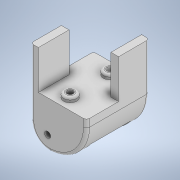
# Autodesk Inventor part: topMountThick
Saved by Autodesk Inventor 2020 (Build 240168000, 168)
## iProperties
Created: 2020-07-25
Part Number: topMountThick
Material: Generic
Document SubType Name: Modeling
Designer: PAB
Density: 1 g/cm^3
Appearance: Default
Author: PAB
Autodesk Inventor part; units mm, degrees
ref_plane "YZ Plane" through (0, 0, 0) normal (1, 0, 0) x (0, 1, 0)
ref_plane "XZ Plane" through (0, 0, 0) normal (0, 1, 0) x (-1, 0, 0)
ref_plane "XY Plane" through (0, 0, 0) normal (0, 0, 1) x (1, 0, 0)
sketch "Sketch1" plane through (0, 0, 0) normal (0, 1, 0) x (-1, 0, 0)
  line L0 (19.2, 20.5) -> (-17.2, 20.5)
  line L1 (-17.2, 20.5) -> (-17.2, -20.5)
  line L2 (-17.2, -20.5) -> (19.2, -20.5)
  line L3 (19.2, -20.5) -> (19.2, 20.5)
  point P0 (0, 0)
  dimension "d0" = 36.4
  dimension "d1" = 41
  constraints: 8 end point, 2 parallel, 1 horizontal, 1 perpendicular
  measures "d0" distance of L2.end L1.end
  measures "d1" distance of L1.end L0.end
extrude "Extrusion1" add sketch "Sketch1" along normal blind 5
sketch "Sketch2" plane through (0, 5, 0) normal (0, 1, 0) x (1, 0, 0)
  line L0 (-19.2, -20.5) -> (17.2, -20.5) projected
  line L1 (-19.2, -20.5) -> (-14.2, -20.5)
  line L2 (-14.2, -20.5) -> (-14.2, -0.5)
  line L3 (-14.2, -0.5) -> (-19.2, -0.5)
  line L4 (-19.2, -0.5) -> (-19.2, -20.5)
  line L5 (17.2, 20.5) -> (-19.2, 20.5) projected
  line L6 (17.2, 20.5) -> (12.2, 20.5)
  line L7 (12.2, 20.5) -> (12.2, 0.5)
  line L8 (12.2, 0.5) -> (17.2, 0.5)
  line L9 (17.2, 0.5) -> (17.2, 20.5)
  point P0 (0, 0)
  dimension "d4" = 5
  dimension "d5" = 20
  dimension "d6" = 5
  dimension "d7" = 20
  constraints: 16 end point, 4 parallel, 2 horizontal, 2 perpendicular
  measures "d4" distance of L3.end L2.end
  measures "d5" distance of L2.end L1.end
  measures "d6" distance of L8.end L7.end
  measures "d7" distance of L7.end L6.end
extrude "Extrusion2" add sketch "Sketch2" along normal blind 25.4
sketch "Sketch3" plane through (0, 5, 0) normal (0, 1, 0) x (1, 0, 0)
  circle A0 centre (-1, -13) radius 4.25
  circle A1 centre (-1, 13) radius 4.25
  line L0 (-14.2, -20.5) -> (-14.2, -0.5) projected
  line L1 (12.2, 20.5) -> (12.2, 0.5) projected
  point P0 (0, 0)
  dimension "d10" = 8.5
  dimension "d11" = 8.5
  dimension "d44" = 13.2
  dimension "d45" = 13.2
  constraints: 2 centre point
  measures "d10" diameter of A0
  measures "d11" diameter of A1
  measures "d44" distance from line of L0 A0.centre
  measures "d45" distance from line of L1 A1.centre
extrude "Extrusion3" add sketch "Sketch3" along normal blind 3
sketch "Sketch4" plane through (-1, 8, 13) normal (0, 1, 0) x (1, 0, 0)
  circle A0 centre (0, 0) radius 4.25 projected
  circle A1 centre (0, 0) radius 2
  circle A2 centre (0, 26) radius 4.25 projected
  circle A3 centre (0, 26) radius 2
  point P0 (1, 13)
  dimension "d14" = 4
  dimension "d15" = 4
  constraints: 2 centre point, 2 coincident
  measures "d14" diameter of A1
  measures "d15" diameter of A3
extrude "Extrusion4" cut sketch "Sketch4" against normal blind 10 contours A1 | A3
fillet "Fillet2" radius 1.5 2 edges at (-5.25, 8, -13) (-5.25, 8, 13)
sketch "Sketch5" plane through (0, 0, 0) normal (0, -1, 0) x (1, 0, 0)
  circle A0 centre (-1, 13) radius 2 projected
  circle A1 centre (-1, 13) radius 3
  circle A2 centre (-1, -13) radius 2 projected
  circle A3 centre (-1, -13) radius 3
  point P0 (0, 0)
  dimension "d20" = 6
  dimension "d21" = 6
  constraints: 2 centre point, 2 coincident
  measures "d20" diameter of A1
  measures "d21" diameter of A3
extrude "Extrusion5" cut sketch "Sketch5" against normal blind 3 contours A0 | A1 | A2 | A3
sketch "Sketch6" plane through (0, 0, 0) normal (0, -1, 0) x (1, 0, 0)
  line L0 (17.2, 20.5) -> (17.2, -20.5) projected
  line L1 (-19.2, -20.5) -> (-19.2, 20.5) projected
  line L2 (17.2, -20.5) -> (-19.2, -20.5)
  line L3 (-19.2, -20.5) -> (-19.2, 20.5)
  line L4 (-19.2, 20.5) -> (17.2, 20.5)
  line L5 (17.2, 20.5) -> (17.2, -20.5)
  point P0 (0, 0)
  constraints: 8 end point, 2 parallel, 1 horizontal, 1 perpendicular
extrude "Extrusion6" add sketch "Sketch6" along normal blind 25
sketch "Sketch7" plane through (0, -25, 0) normal (0, -1, 0) x (1, 0, 0)
  line L0 (-19.2, -13) -> (-4.2, -13)
  line L1 (-4.2, -13) -> (-4.2, -9.525)
  line L2 (-4.2, -9.525) -> (-19.2, -9.525)
  line L3 (-19.2, -9.525) -> (-19.2, -13)
  point P0 (0, 0)
  dimension "d26" = 15
  constraints: 8 end point, 2 parallel, 1 horizontal, 1 perpendicular
  measures "d26" distance of L2.end L1.end
extrude "Extrusion7" cut sketch "Sketch7" against normal blind 15
sketch "Sketch8" plane through (-19.2, -25, -13) normal (0, 0, 1) x (1, 0, 0)
  circle A0 centre (11, 9) radius 15.5
  point P0 (19.2, 25)
  dimension "d29" = 31
  constraints: 1 centre point
  measures "d29" diameter of A0
extrude "Extrusion8" cut sketch "Sketch8" along normal blind 26
sketch "Sketch9" plane through (-19.2, -25, -13) normal (0, 0, 1) x (1, 0, 0)
  arc A0 (23.6194, 0) -> (0, 19.9202) centre (11, 9) ccw projected
  circle A1 centre (11, 9) radius 2
  point P0 (19.2, 25)
  dimension "d32" = 4
  constraints: 1 centre point, 1 coincident
  measures "d32" diameter of A1
extrude "Extrusion9" cut sketch "Sketch9" against normal mid plane 100
fillet "Fillet3" radius 25 1 edges at (17.2, -25, 0)
fillet "Fillet4" radius 3 1 edges at (6.6653, -20.3901, 0)
fillet "Fillet5" radius 12 2 edges at (-19.2, -25, -16.75) (-19.2, -25, 16.75)
fillet "Fillet6" radius 2 1 edges at (-19.2, -5.0798, 0)
fillet "Fillet7" radius 2 8 edges at (17.2, 15.2, -20.5) (-15.4872, -21.665, -20.5) (-19.2, -3.9931, -20.5) (10.281, -17.2649, -20.5) (-15.4872, -21.665, 20.5) (-19.2, 8.7069, 20.5) (17.2, 2.5, 20.5) (10.281, -17.2649, 20.5)
sketch "Sketch10" plane through (-1, 0, -13) normal (0, 1, 0) x (1, 0, 0)
  circle A0 centre (0, 0) radius 3 projected
  circle A1 centre (0, 0) radius 3
  circle A2 centre (0, -26) radius 2 projected
  circle A3 centre (0, -26) radius 3
  point P0 (1, -13)
  dimension "d40" = 6
  dimension "d41" = 6
  constraints: 2 centre point, 2 coincident
  measures "d40" diameter of A1
  measures "d41" diameter of A3
extrude "Extrusion10" cut sketch "Sketch10" against normal blind 30 contours A0 | A2 | A3
body "Solid1"
